Autodesk Fusion 360 part; units mm, degrees
note: some values were not read from the file. Chosen so that the rebuilt part matches the saved one: which bodies a step acts on. Set by a fixed rule: which sketch regions a step uses.
(part 2 of 2)
sketch "Sketch36" plane through (-3.3, 0, 0) normal (-1, 0, 0) x (0, -1, 0)
  line L0 (50, 42.2) -> (57.6, 42.2)
  line L1 (57.6, 42.2) -> (57.6, 27.6)
  line L2 (57.6, 27.6) -> (50, 27.6)
  line L3 (50, 27.6) -> (50, 22.6)
  line L4 (50, 22.6) -> (57.5, 22.6)
  line L5 (57.5, 22.6) -> (57.5, 8)
  line L6 (57.5, 8) -> (50, 8)
  line L7 (50, 8) -> (50, 4)
  line L8 (50, 4) -> (75, 4)
  line L9 (75, 4) -> (75, 53)
  line L10 (75, 53) -> (50, 53)
  line L11 (50, 53) -> (50, 49.75)
  line L12 (50, 49.75) -> (52, 49.75)
  line L13 (52, 49.75) -> (52, 46.25)
  line L14 (52, 46.25) -> (50, 46.25)
  line L15 (50, 46.25) -> (50, 42.2)
extrude "Extrude59" add 2 faces at (53.0448, -67, 50.2683) (4.0448, -67, 50.2683) along direction (0, 1, 0) blind 1 on bodies 3 bodies 3
extrude "Extrude60" cut 2 faces at (54.0333, -55.3333, 56.1) (2.9667, -55.3333, 56.1) along direction (0, 0, -1) blind 55.1 on bodies 3 bodies 3
sketch "Sketch37" plane through (0, -66, 0) normal (0, 1, 0) x (-1, 0, 0)
  circle A0 centre (-4, 53) radius 1.8
  line L0 (-0.9, 49.8) -> (-0.9, 56.1)
  line L1 (-0.9, 56.1) -> (-7.1, 56.1)
  line L2 (-7.1, 56.1) -> (-7.1, 49.8)
  line L3 (-7.1, 49.8) -> (-0.9, 49.8)
sketch "Sketch38" plane through (0, -66, 0) normal (0, 1, 0) x (-1, 0, 0)
  circle A0 centre (-4, 53) radius 1.8
  line L0 (-0.9, 49.8) -> (-0.9, 56.1)
  line L1 (-0.9, 56.1) -> (-7.1, 56.1)
  line L2 (-7.1, 56.1) -> (-7.1, 49.8)
  line L3 (-7.1, 49.8) -> (-0.9, 49.8)
sketch "Sketch39" plane through (0, -50, 0) normal (0, 1, 0) x (-1, 0, 0)
  line L0 (-49.9, 7.2) -> (-49.9, 1)
  line L1 (-49.9, 1) -> (-56.1, 1)
  line L2 (-56.1, 1) -> (-56.1, 7.2)
  line L3 (-56.1, 7.2) -> (-57.8, 7.2)
  line L4 (-57.8, 7.2) -> (-57.8, 15.95)
  line L5 (-57.8, 15.95) -> (-60.3, 15.95)
  line L6 (-60.3, 15.95) -> (-60.3, 4)
  arc A0 (-60.3, 4) -> (-53, -3.3) centre (-53, 4) ccw
  line L7 (-53, -3.3) -> (-4, -3.3)
  arc A1 (-4, -3.3) -> (3.3, 4) centre (-4, 4) ccw
  line L8 (3.3, 4) -> (3.3, 8)
  line L9 (3.3, 8) -> (0.8, 8)
  line L10 (0.8, 8) -> (0.8, 7.2)
  line L11 (0.8, 7.2) -> (-0.9, 7.2)
  line L12 (-0.9, 7.2) -> (-0.9, 1)
  line L13 (-0.9, 1) -> (-7.1, 1)
  line L14 (-7.1, 1) -> (-7.1, 7.2)
  line L15 (-7.1, 7.2) -> (-7.2, 7.2)
  line L16 (-7.2, 7.2) -> (-7.2, -0.8)
  line L17 (-7.2, -0.8) -> (-49.8, -0.8)
  line L18 (-49.8, -0.8) -> (-49.8, 7.2)
  line L19 (-49.8, 7.2) -> (-49.9, 7.2)
  line L20 (-0.9, 1) -> (-7.1, 1)
  line L21 (-7.1, 1) -> (-7.1, 7.2)
  line L22 (-7.1, 7.2) -> (-0.9, 7.2)
  line L23 (-0.9, 7.2) -> (-0.9, 1)
  line L24 (-56.1, 1) -> (-49.8, 1)
  line L25 (-49.8, 1) -> (-49.8, 7.2)
  line L26 (-49.8, 7.2) -> (-56.1, 7.2)
  line L27 (-56.1, 7.2) -> (-56.1, 1)
  line L28 (-0.9, 1) -> (-7.2, 1)
  line L29 (-7.2, 1) -> (-7.2, 7.2)
  line L30 (-7.2, 7.2) -> (-0.9, 7.2)
  line L31 (-0.9, 7.2) -> (-0.9, 1)
  constraint horizontal L20
  constraint vertical L21
  constraint horizontal L22
  constraint vertical L23
  constraint coincident L14.end L15.start
  constraint coincident L12.end L13.start
  constraint horizontal L24
  constraint vertical L25
  constraint horizontal L26
  constraint vertical L27
  constraint coincident L18.end L19.start
  constraint coincident L1.end L2.start
  constraint horizontal L28
  constraint vertical L29
  constraint horizontal L30
  constraint vertical L31
  constraint coincident L15.end L16.start
extrude "Extrude61" add sketch "Sketch39" against normal blind 13 contours L0 L18 L19 L24 L25 L26 | L0 L1 L2 L24 L26 L27 | L14 L15 L16 L21 L28 L29 L30 | L12 L13 L14 L20 L21 L22 L23 L28 L30 L31 bodies 3
sketch "Sketch40" plane through (0, -50, 0) normal (0, 1, 0) x (-1, 0, 0)
  line L0 (-0.9, 56.1) -> (-0.9, 49.8)
  line L1 (-0.9, 49.8) -> (0.8, 49.8)
  line L2 (0.8, 49.8) -> (0.8, 49.75)
  line L3 (0.8, 49.75) -> (3.3, 49.75)
  line L4 (3.3, 49.75) -> (3.3, 53)
  arc A0 (3.3, 53) -> (-4, 60.3) centre (-4, 53) ccw
  line L5 (-4, 60.3) -> (-53, 60.3)
  arc A1 (-53, 60.3) -> (-60.3, 53) centre (-53, 53) ccw
  line L6 (-60.3, 53) -> (-60.3, 19.45)
  line L7 (-60.3, 19.45) -> (-57.8, 19.45)
  line L8 (-57.8, 19.45) -> (-57.8, 49.8)
  line L9 (-57.8, 49.8) -> (-56.1, 49.8)
  line L10 (-56.1, 49.8) -> (-56.1, 56.1)
  line L11 (-56.1, 56.1) -> (-49.9, 56.1)
  line L12 (-49.9, 56.1) -> (-49.9, 49.8)
  line L13 (-49.9, 49.8) -> (-49.8, 49.8)
  line L14 (-49.8, 49.8) -> (-49.8, 57.8)
  line L15 (-49.8, 57.8) -> (-7.2, 57.8)
  line L16 (-7.2, 57.8) -> (-7.2, 49.8)
  line L17 (-7.2, 49.8) -> (-7.1, 49.8)
  line L18 (-7.1, 49.8) -> (-7.1, 56.1)
  line L19 (-7.1, 56.1) -> (-0.9, 56.1)
  line L20 (-56.1, 56.1) -> (-49.9, 56.1)
  line L21 (-49.9, 56.1) -> (-49.9, 49.8)
  line L22 (-49.9, 49.8) -> (-56.1, 49.8)
  line L23 (-56.1, 49.8) -> (-56.1, 56.1)
  line L24 (-0.9, 56.1) -> (-7.1, 56.1)
  line L25 (-7.1, 56.1) -> (-7.1, 49.8)
  line L26 (-7.1, 49.8) -> (-0.9, 49.8)
  line L27 (-0.9, 49.8) -> (-0.9, 56.1)
  constraint horizontal L20
  constraint vertical L21
  constraint horizontal L22
  constraint vertical L23
  constraint coincident L12.end L13.start
  constraint coincident L10.end L11.start
  constraint horizontal L24
  constraint vertical L25
  constraint horizontal L26
  constraint vertical L27
  constraint coincident L17.end L18.start
  constraint coincident L0.start L19.end
extrude "Extrude62" add sketch "Sketch40" against normal blind 13 contours L0 L18 L19 L24 L25 L26 L27 | L10 L11 L12 L20 L21 L22 L23 bodies 3
sketch "Sketch41" plane through (0, -77.5, 0) normal (0, -1, 0) x (1, 0, 0)
  circle A0 centre (4, 4) radius 1.8
  circle A1 centre (4, 53) radius 1.8
  circle A2 centre (53, 4) radius 1.8
  circle A3 centre (53, 53) radius 1.8
  circle A4 centre (39, 43.5) radius 6
  circle A5 centre (18, 43.5) radius 7
  arc A6 (-0.8, 4) -> (4, -0.8) centre (4, 4) ccw
  line L0 (4, -0.8) -> (53, -0.8)
  arc A7 (53, -0.8) -> (57.8, 4) centre (53, 4) ccw
  line L1 (57.8, 4) -> (57.8, 53)
  arc A8 (57.8, 53) -> (53, 57.8) centre (53, 53) ccw
  line L2 (53, 57.8) -> (4, 57.8)
  arc A9 (4, 57.8) -> (-0.8, 53) centre (4, 53) ccw
  line L3 (-0.8, 53) -> (-0.8, 4)
extrude "Extrude63" add sketch "Sketch41" against normal blind 3 contours A0 | A1 | A2 | A3 bodies 3
sketch "Sketch42" plane through (0, -75, 0) normal (0, 1, 0) x (-1, 0, 0)
  arc A0 (-41.1817, 55.3) -> (-27.4524, 40.2362) centre (-39, 43.5) ccw
  line L0 (-41.1817, 55.3) -> (-49.8, 55.3)
  line L1 (-49.8, 55.3) -> (-49.8, 49.8)
  line L2 (-49.8, 49.8) -> (-55.3, 49.8)
  line L3 (-55.3, 49.8) -> (-55.3, 7.2)
  line L4 (-55.3, 7.2) -> (-49.8, 7.2)
  line L5 (-49.8, 7.2) -> (-49.8, 1.7)
  line L6 (-49.8, 1.7) -> (-7.2, 1.7)
  line L7 (-7.2, 1.7) -> (-7.2, 7.2)
  line L8 (-7.2, 7.2) -> (-1.7, 7.2)
  line L9 (-1.7, 7.2) -> (-1.7, 49.8)
  line L10 (-1.7, 49.8) -> (-7.2, 49.8)
  line L11 (-7.2, 49.8) -> (-7.2, 55.3)
  line L12 (-7.2, 55.3) -> (-36.8183, 55.3)
  arc A1 (-27.4524, 46.7638) -> (-36.8183, 55.3) centre (-39, 43.5) ccw
  arc A2 (-27.4524, 40.2362) -> (-27.4524, 46.7638) centre (-18, 43.5) ccw
  line L13 (-7.2, 49.8) -> (-9.2, 49.8)
  line L14 (-9.2, 49.8) -> (-9.2, 58.8)
  line L15 (-9.2, 58.8) -> (-7.2, 58.8)
  line L16 (-7.2, 58.8) -> (-7.2, 49.8)
  line L17 (-49.8, 49.8) -> (-47.8, 49.8)
  line L18 (-47.8, 49.8) -> (-47.8, 58.8)
  line L19 (-47.8, 58.8) -> (-49.8, 58.8)
  line L20 (-49.8, 58.8) -> (-49.8, 49.8)
  dimension "d264" = 2
  dimension "d265" = 9
  dimension "d266" = 2
  dimension "d267" = 9
  constraint horizontal L13
  constraint vertical L14
  constraint horizontal L15
  constraint vertical L16
  constraint coincident L10.end L11.start
  constraint horizontal L17
  constraint vertical L18
  constraint horizontal L19
  constraint vertical L20
  constraint coincident L1.end L2.start
  measures "d264" distance of L10.end L13.end
  measures "d265" distance of L10.end L15.end
  measures "d266" distance of L1.end L17.end
  measures "d267" distance of L1.end L19.end
extrude "Extrude64" add sketch "Sketch42" along normal blind 13 contours A0 L17 L18 | A0 L0 L1 L17 L18 L20 | L0 L18 L19 L20 | L12 L14 L15 L16 | L11 L12 L13 L14 L16 bodies 3
sketch "Sketch43" plane through (0, -75, 0) normal (0, 1, 0) x (-1, 0, 0)
  line L0 (-1.7, 49.8) -> (-9.2, 49.8)
  line L1 (-9.2, 49.8) -> (-9.2, 55.3)
  line L2 (-9.2, 55.3) -> (-36.8183, 55.3)
  arc A0 (-27.4524, 46.7638) -> (-36.8183, 55.3) centre (-39, 43.5) ccw
  arc A1 (-27.4524, 40.2362) -> (-27.4524, 46.7638) centre (-18, 43.5) ccw
  arc A2 (-49.2132, 49.8) -> (-27.4524, 40.2362) centre (-39, 43.5) ccw
  line L3 (-49.2132, 49.8) -> (-55.3, 49.8)
  line L4 (-55.3, 49.8) -> (-55.3, 7.2)
  line L5 (-55.3, 7.2) -> (-49.8, 7.2)
  line L6 (-49.8, 7.2) -> (-49.8, 1.7)
  line L7 (-49.8, 1.7) -> (-7.2, 1.7)
  line L8 (-7.2, 1.7) -> (-7.2, 7.2)
  line L9 (-7.2, 7.2) -> (-1.7, 7.2)
  line L10 (-1.7, 7.2) -> (-1.7, 49.8)
  line L11 (-7.2, 7.2) -> (-9.2, 7.2)
  line L12 (-9.2, 7.2) -> (-9.2, -1.8)
  line L13 (-9.2, -1.8) -> (-7.2, -1.8)
  line L14 (-7.2, -1.8) -> (-7.2, 7.2)
  line L15 (-49.8, 7.2) -> (-47.8, 7.2)
  line L16 (-47.8, 7.2) -> (-47.8, -1.8)
  line L17 (-47.8, -1.8) -> (-49.8, -1.8)
  line L18 (-49.8, -1.8) -> (-49.8, 7.2)
  dimension "d270" = 2
  dimension "d271" = 9
  dimension "d272" = 2
  dimension "d273" = 9
  constraint horizontal L11
  constraint vertical L12
  constraint horizontal L13
  constraint vertical L14
  constraint coincident L8.end L9.start
  constraint horizontal L15
  constraint vertical L16
  constraint horizontal L17
  constraint vertical L18
  constraint coincident L5.end L6.start
  measures "d270" distance of L8.end L11.end
  measures "d271" distance of L8.end L13.end
  measures "d272" distance of L5.end L15.end
  measures "d273" distance of L5.end L17.end
extrude "Extrude65" add sketch "Sketch43" along normal blind 13 contours L7 L8 L11 L12 L14 | L7 L12 L13 L14 | L7 L16 L17 L18 | L6 L7 L15 L16 L18 bodies 3
sketch "Sketch44" plane through (0, 1.25, 0) normal (0, -1, 0) x (1, 0, 0)
  circle A0 centre (4, 4) radius 1.8
  circle A1 centre (4, 53) radius 1.8
  circle A2 centre (53, 4) radius 1.8
  circle A3 centre (53, 53) radius 1.8
  line L0 (21.9074, 57.8) -> (21.9074, 55.8)
  line L1 (21.9074, 55.8) -> (49.8, 55.8)
  line L2 (49.8, 55.8) -> (49.8, 49.8)
  line L3 (49.8, 49.8) -> (55.8, 49.8)
  line L4 (55.8, 49.8) -> (55.8, 7.2)
  line L5 (55.8, 7.2) -> (49.8, 7.2)
  line L6 (49.8, 7.2) -> (49.8, 1.2)
  line L7 (49.8, 1.2) -> (7.2, 1.2)
  line L8 (7.2, 1.2) -> (7.2, 7.2)
  line L9 (7.2, 7.2) -> (1.2, 7.2)
  line L10 (1.2, 7.2) -> (1.2, 49.8)
  line L11 (1.2, 49.8) -> (7.2, 49.8)
  line L12 (7.2, 49.8) -> (7.2, 57.8)
  line L13 (7.2, 57.8) -> (4, 57.8)
  arc A4 (4, 57.8) -> (-0.8, 53) centre (4, 53) ccw
  line L14 (-0.8, 53) -> (-0.8, 4)
  arc A5 (-0.8, 4) -> (4, -0.8) centre (4, 4) ccw
  line L15 (4, -0.8) -> (53, -0.8)
  arc A6 (53, -0.8) -> (57.8, 4) centre (53, 4) ccw
  line L16 (57.8, 4) -> (57.8, 53)
  arc A7 (57.8, 53) -> (53, 57.8) centre (53, 53) ccw
  line L17 (53, 57.8) -> (21.9074, 57.8)
sketch "Sketch45" plane through (0, 1.25, 0) normal (0, -1, 0) x (1, 0, 0)
  circle A0 centre (4, 4) radius 1.8
  circle A1 centre (4, 53) radius 1.8
  circle A2 centre (53, 4) radius 1.8
  circle A3 centre (53, 53) radius 1.8
  line L0 (21.9074, 57.8) -> (21.9074, 55.8)
  line L1 (21.9074, 55.8) -> (49.8, 55.8)
  line L2 (49.8, 55.8) -> (49.8, 49.8)
  line L3 (49.8, 49.8) -> (55.8, 49.8)
  line L4 (55.8, 49.8) -> (55.8, 7.2)
  line L5 (55.8, 7.2) -> (49.8, 7.2)
  line L6 (49.8, 7.2) -> (49.8, 1.2)
  line L7 (49.8, 1.2) -> (7.2, 1.2)
  line L8 (7.2, 1.2) -> (7.2, 7.2)
  line L9 (7.2, 7.2) -> (1.2, 7.2)
  line L10 (1.2, 7.2) -> (1.2, 49.8)
  line L11 (1.2, 49.8) -> (7.2, 49.8)
  line L12 (7.2, 49.8) -> (7.2, 57.8)
  line L13 (7.2, 57.8) -> (4, 57.8)
  arc A4 (4, 57.8) -> (-0.8, 53) centre (4, 53) ccw
  line L14 (-0.8, 53) -> (-0.8, 4)
  arc A5 (-0.8, 4) -> (4, -0.8) centre (4, 4) ccw
  line L15 (4, -0.8) -> (53, -0.8)
  arc A6 (53, -0.8) -> (57.8, 4) centre (53, 4) ccw
  line L16 (57.8, 4) -> (57.8, 53)
  arc A7 (57.8, 53) -> (53, 57.8) centre (53, 53) ccw
  line L17 (53, 57.8) -> (21.9074, 57.8)
sketch "Sketch46" plane through (0, 1.25, 0) normal (0, -1, 0) x (1, 0, 0)
  circle A0 centre (4, 4) radius 1.8
  circle A1 centre (4, 53) radius 1.8
  circle A2 centre (53, 4) radius 1.8
  circle A3 centre (53, 53) radius 1.8
  line L0 (21.9074, 57.8) -> (21.9074, 55.8)
  line L1 (21.9074, 55.8) -> (49.8, 55.8)
  line L2 (49.8, 55.8) -> (49.8, 49.8)
  line L3 (49.8, 49.8) -> (55.8, 49.8)
  line L4 (55.8, 49.8) -> (55.8, 7.2)
  line L5 (55.8, 7.2) -> (49.8, 7.2)
  line L6 (49.8, 7.2) -> (49.8, 1.2)
  line L7 (49.8, 1.2) -> (7.2, 1.2)
  line L8 (7.2, 1.2) -> (7.2, 7.2)
  line L9 (7.2, 7.2) -> (1.2, 7.2)
  line L10 (1.2, 7.2) -> (1.2, 49.8)
  line L11 (1.2, 49.8) -> (7.2, 49.8)
  line L12 (7.2, 49.8) -> (7.2, 57.8)
  line L13 (7.2, 57.8) -> (4, 57.8)
  arc A4 (4, 57.8) -> (-0.8, 53) centre (4, 53) ccw
  line L14 (-0.8, 53) -> (-0.8, 4)
  arc A5 (-0.8, 4) -> (4, -0.8) centre (4, 4) ccw
  line L15 (4, -0.8) -> (53, -0.8)
  arc A6 (53, -0.8) -> (57.8, 4) centre (53, 4) ccw
  line L16 (57.8, 4) -> (57.8, 53)
  arc A7 (57.8, 53) -> (53, 57.8) centre (53, 53) ccw
  line L17 (53, 57.8) -> (21.9074, 57.8)
  circle A8 centre (4, 4) radius 1.55
  circle A9 centre (53, 4) radius 1.55
  circle A10 centre (53, 53) radius 1.55
  circle A11 centre (4, 53) radius 1.55
  circle A12 centre (53, 53) radius 1.8
  circle A13 centre (4, 53) radius 1.8
  circle A14 centre (4, 4) radius 1.8
  circle A15 centre (53, 4) radius 1.8
  dimension "d276" = 3.1
  dimension "d277" = 3.1
  dimension "d278" = 3.1
  dimension "d279" = 3.1
  constraint concentric A0 A8
  constraint concentric A2 A9
  constraint concentric A3 A10
  constraint concentric A1 A11
  constraint concentric A3 A12
  constraint concentric A1 A13
  constraint concentric A0 A14
  constraint concentric A9 A15
  measures "d276" diameter of A8
  measures "d277" diameter of A9
  measures "d278" diameter of A10
  measures "d279" diameter of A11
extrude "Extrude66" add sketch "Sketch46" against normal blind 6.25 contours A0 A14 | A1 A13 | A2 A15 | A3 A12 bodies 2
sketch "Sketch47" plane through (0, 12.5, 0) normal (0, 1, 0) x (-1, 0, 0)
  circle A0 centre (-4, 53) radius 3.25
  circle A1 centre (-4, 4) radius 3.25
  circle A2 centre (-53, 53) radius 3.25
  circle A3 centre (-53, 4) radius 3.25
  line L0 (-4, 60.3) -> (-53, 60.3)
  arc A4 (-53, 60.3) -> (-60.3, 53) centre (-53, 53) ccw
  line L1 (-60.3, 53) -> (-60.3, 4)
  arc A5 (-60.3, 4) -> (-53, -3.3) centre (-53, 4) ccw
  line L2 (-53, -3.3) -> (-4, -3.3)
  arc A6 (-4, -3.3) -> (3.3, 4) centre (-4, 4) ccw
  line L3 (3.3, 4) -> (3.3, 53)
  arc A7 (3.3, 53) -> (-4, 60.3) centre (-4, 53) ccw
  circle A8 centre (-4, 4) radius 1.55
  circle A9 centre (-53, 4) radius 1.55
  circle A10 centre (-53, 53) radius 1.55
  circle A11 centre (-4, 53) radius 1.55
  dimension "d282" = 3.1
  dimension "d283" = 3.1
  dimension "d284" = 3.1
  dimension "d285" = 3.1
  constraint concentric A1 A8
  constraint concentric A3 A9
  constraint concentric A2 A10
  constraint concentric A0 A11
  measures "d282" diameter of A8
  measures "d283" diameter of A9
  measures "d284" diameter of A10
  measures "d285" diameter of A11
extrude "Extrude67" cut sketch "Sketch47" against normal blind 77 contours A8 | A9 | A10 | A11 bodies 3
extrude "Extrude68" add 1 faces at (31.0558, -65, 42.7548) along direction (0, 1, 0) blind 8 on bodies 3 bodies 3
sketch "Sketch48" plane through (0, -57, 0) normal (0, 1, 0) x (-1, 0, 0)
  circle A0 centre (-39, 43.5) radius 9
  circle A1 centre (-39, 43.5) radius 6
  circle A2 centre (-39, 43.5) radius 6
  constraint concentric A0 A2
extrude "Extrude69" add sketch "Sketch48" against normal blind 2 contours A1 A2 bodies 3
sketch "Sketch49" plane through (0, -59, 0) normal (0, -1, 0) x (1, 0, 0)
  circle A0 centre (39, 43.5) radius 6
  circle A1 centre (39, 43.5) radius 3.5
  circle A2 centre (39, 43.5) radius 2.369
  dimension "d292" = 7
  constraint concentric A0 A1
  constraint concentric A1 A2
  measures "d292" diameter of A1
extrude "Extrude70" cut sketch "Sketch49" against normal blind 4 contours A1 | A2 bodies 3
fillet "Fillet8" radius 5.5 1 edges at (33.406, -59, 45.6697) on bodies 3
fillet "Fillet9" radius 1.5 1 edges at (7.2, -62, 53.8) on bodies 3
fillet "Fillet10" radius 2 3 edges at (49.8, -62, 53.8) (49.8, -62, 3.2) (7.2, -62, 3.2) on bodies 3
sketch "Sketch50" plane through (0, -77.5, 0) normal (0, -1, 0) x (1, 0, 0)
  circle A0 centre (39, 43.5) radius 6
  circle A1 centre (18, 43.5) radius 7
  arc A2 (-0.8, 4) -> (4, -0.8) centre (4, 4) ccw
  line L0 (4, -0.8) -> (53, -0.8)
  arc A3 (53, -0.8) -> (57.8, 4) centre (53, 4) ccw
  line L1 (57.8, 4) -> (57.8, 53)
  arc A4 (57.8, 53) -> (53, 57.8) centre (53, 53) ccw
  line L2 (53, 57.8) -> (4, 57.8)
  arc A5 (4, 57.8) -> (-0.8, 53) centre (4, 53) ccw
  line L3 (-0.8, 53) -> (-0.8, 4)
extrude "Extrude71" add sketch "Sketch50" along normal blind 15 separate body contours A1 makes body 6
sketch "Sketch51" plane through (0, -92.5, 0) normal (0, -1, 0) x (1, 0, 0)
  circle A0 centre (18, 43.5) radius 7
  circle A1 centre (18, 43.5) radius 1.3957
  circle A2 centre (18, 43.5) radius 3.297
  constraint concentric A0 A1
  constraint concentric A1 A2
extrude "Extrude72" cut sketch "Sketch51" against normal blind 11 contours A1 | A2 bodies 6
move_body "Move3" bodies 1 to x (1, 0, 0) y (0, 1, 0) z (0, 0, 1) at (0, 20, 0)
move_body "Move4" bodies 3 to x (1, 0, 0) y (0, 1, 0) z (0, 0, 1) at (0, 50, 0)
move_body "Move5" bodies 6 to x (1, 0, 0) y (0, 1, 0) z (0, 0, 1) at (0, 50, 0)
sketch "Sketch52" plane through (0, 0, 60.3) normal (0, 0, 1) x (-1, 0, 0)
  circle A0 centre (-11.43, 8.81) radius 3
  line L0 (-4, 25) -> (-53, 25)
  line L1 (-53, 25) -> (-53, 0)
  line L2 (-53, 0) -> (-4, 0)
  line L3 (-4, 0) -> (-4, 25)
extrude "Extrude73" add sketch "Sketch52" along normal blind 10 separate body contours A0 makes body 7
sketch "Sketch53" plane through (0, -31.5, 0) normal (0, -1, 0) x (1, 0, 0)
  circle A0 centre (18, 43.5) radius 3.297
  circle A1 centre (18, 43.5) radius 2.7993
  constraint concentric A0 A1
extrude "Extrude74" add sketch "Sketch53" 1 faces at (16.4003, -31.5, 44.3672) along normal blind 6 contours A1 on bodies 6 bodies 6
sketch "Sketch54" plane through (0, 9.5, 0) normal (0, -1, 0) x (1, 0, 0)
  line L0 (9.7, 9.7) -> (9.7, 1.2)
  line L1 (9.7, 1.2) -> (47.3, 1.2)
  line L2 (47.3, 1.2) -> (47.3, 9.7)
  line L3 (47.3, 9.7) -> (55.8, 9.7)
  line L4 (55.8, 9.7) -> (55.8, 47.3)
  line L5 (55.8, 47.3) -> (47.3, 47.3)
  line L6 (47.3, 47.3) -> (47.3, 55.8)
  line L7 (47.3, 55.8) -> (9.7, 55.8)
  line L8 (9.7, 55.8) -> (9.7, 47.3)
  line L9 (9.7, 47.3) -> (1.2, 47.3)
  line L10 (1.2, 47.3) -> (1.2, 9.7)
  line L11 (1.2, 9.7) -> (9.7, 9.7)
  circle A0 centre (38.9991, 43.5419) radius 3.0067
extrude "Extrude75" add sketch "Sketch49" along normal blind 6 contours A2 bodies 3 makes body 8
move_body "Move6" bodies 8 to x (1, 0, 0) y (0, 1, 0) z (0, 0, 1) at (0, 59, 0)
sketch "Sketch55" plane through (-3.3, 0, 0) normal (-1, 0, 0) x (0, -1, 0)
  line L0 (0, 42.2) -> (7.6, 42.2)
  line L1 (7.6, 42.2) -> (7.6, 27.6)
  line L2 (7.6, 27.6) -> (0, 27.6)
  line L3 (0, 27.6) -> (0, 22.6)
  line L4 (0, 22.6) -> (7.5, 22.6)
  line L5 (7.5, 22.6) -> (7.5, 8)
  line L6 (7.5, 8) -> (0, 8)
  line L7 (0, 8) -> (0, 4)
  line L8 (0, 4) -> (25, 4)
  line L9 (25, 4) -> (25, 53)
  line L10 (25, 53) -> (0, 53)
  line L11 (0, 53) -> (0, 49.75)
  line L12 (0, 49.75) -> (2, 49.75)
  line L13 (2, 49.75) -> (2, 46.25)
  line L14 (2, 46.25) -> (0, 46.25)
  line L15 (0, 46.25) -> (0, 42.2)
  line L16 (0, 42) -> (7.6, 42)
  line L17 (7.6, 42) -> (7.6, 27.6)
  line L18 (7.6, 27.6) -> (0, 27.6)
  line L19 (0, 27.6) -> (0, 42)
  line L20 (0.4121, 22.6) -> (7.5, 22.6)
  line L21 (7.5, 22.6) -> (7.5, 8)
  line L22 (7.5, 8) -> (0.4121, 8)
  line L23 (0.4121, 8) -> (0.4121, 22.6)
  constraint horizontal L16
  constraint vertical L17
  constraint horizontal L18
  constraint vertical L19
  constraint coincident L1.end L2.start
  constraint horizontal L20
  constraint vertical L21
  constraint horizontal L22
  constraint vertical L23
  constraint coincident L5.end L6.start
  constraint coincident L4 L20.start
sketch "Sketch56" plane through (-3.3, 0, 0) normal (-1, 0, 0) x (0, -1, 0)
  line L0 (0, 42.2) -> (7.6, 42.2)
  line L1 (7.6, 42.2) -> (7.6, 27.6)
  line L2 (7.6, 27.6) -> (0, 27.6)
  line L3 (0, 27.6) -> (0, 22.6)
  line L4 (0, 22.6) -> (7.5, 22.6)
  line L5 (7.5, 22.6) -> (7.5, 8)
  line L6 (7.5, 8) -> (0, 8)
  line L7 (0, 8) -> (0, 4)
  line L8 (0, 4) -> (25, 4)
  line L9 (25, 4) -> (25, 53)
  line L10 (25, 53) -> (0, 53)
  line L11 (0, 53) -> (0, 49.75)
  line L12 (0, 49.75) -> (2, 49.75)
  line L13 (2, 49.75) -> (2, 46.25)
  line L14 (2, 46.25) -> (0, 46.25)
  line L15 (0, 46.25) -> (0, 42.2)
extrude "Extrude76" add sketch "Sketch55" along normal blind 0.1 separate body contours L1 L2 L16 L17 L18 L19 | L4 L5 L6 L20 L21 L22 L23 makes body 9 at (-3.3, -2.5333, 37.2) makes body 10 at (-3.3, -2.7747, 12.8667)
copy_body "CopyPasteBodies1" bodies 3 7 10 1 8 6 9 2 makes body 11 makes body 12 makes body 13 makes body 14 makes body 15 makes body 16 makes body 17 makes body 18
move_body "Move7" bodies 11 12 13 14 15 16 17 18 to x (-1, 0, 0) y (0, -1, 0) z (0, 0, 1) at (56.4, -195, 0)
sketch "Sketch57" plane through (0, 0, -3.3) normal (0, 0, -1) x (1, 0, 0)
  line L0 (53, 25) -> (4, 25)
  line L1 (4, 25) -> (4, 0)
  line L2 (4, 0) -> (53, 0)
  line L3 (53, 0) -> (53, 25)
  line L4 (-3.2283, -12.3465) -> (5.4051, -12.3465)
  line L5 (5.4051, -12.3465) -> (5.4051, -51.3017)
  line L6 (5.4051, -51.3017) -> (-3.2283, -51.3017)
  line L7 (-3.2283, -51.3017) -> (-3.2283, -12.3465)
  line L8 (-3.2283, -51.3017) -> (126.4124, -51.3017)
  line L9 (126.4124, -51.3017) -> (126.4124, 265.7054)
  line L10 (126.4124, 265.7054) -> (-3.2283, 265.7054)
  line L11 (-3.2283, 265.7054) -> (-3.2283, -51.3017)
  constraint horizontal L4
  constraint vertical L5
  constraint horizontal L6
  constraint vertical L7
  constraint horizontal L8
  constraint vertical L9
  constraint horizontal L10
  constraint vertical L11
extrude "Extrude77" add sketch "Sketch57" along normal blind 10 contours L4 L5 L8 L9 L10 L11 bodies 2 6 7 9 10 12 13 14 16 17 3 11 18
extrude "Extrude78" add 1 faces at (5.4051, 25.3827, -9.9667) along direction (-1, 0, 0) blind 9 on bodies 2 bodies 2
extrude "Extrude79" cut 1 faces at (-3.3505, 12.3465, -6.6333) along direction (0, 1, 0) blind 62 on bodies 2 bodies 2
split "Split1" by plane through (5.4051, 12.3465, -3.3) normal (0, 0, 1) bodies 2 makes body 19 at (35.2725, -207.5, 21.0702) makes body 20 at (21.1275, 12.5, 21.0702)
extrude "Extrude80" add 1 faces at (126.4124, -54.3673, -6.6333) along direction (1, 0, 0) blind 360 on bodies 2 bodies 2
extrude "Extrude81" add 1 faces at (323.1988, 51.3017, -9.9667) along direction (0, 1, 0) blind 525 on bodies 2 bodies 2
extrude "Extrude82" add 1 faces at (323.1988, -265.7054, -6.6333) along direction (0, -1, 0) blind 340 on bodies 2 bodies 2
move_body "Move8" bodies 2 to x (1, 0, 0) y (0, 1, 0) z (0, 0, 1) at (-170, 0, 0)
extrude "Extrude1" [suppressed]
extrude "Extrude2" [suppressed]
extrude "Extrude3" [suppressed]
sketch "Sketch2" plane through (0, 20, 0) normal (0, 1, 0) x (-1, 0, 0)
  arc A0 (-53, 57.8) -> (-57.8, 53) centre (-53, 53) ccw
  line L0 (-53, 57.8) -> (-4, 57.8)
  arc A1 (0.8, 53) -> (-4, 57.8) centre (-4, 53) ccw
  line L1 (0.8, 53) -> (0.8, 4)
  arc A2 (-4, -0.8) -> (0.8, 4) centre (-4, 4) ccw
  line L2 (-4, -0.8) -> (-53, -0.8)
  arc A3 (-57.8, 4) -> (-53, -0.8) centre (-53, 4) ccw
  line L3 (-57.8, 4) -> (-57.8, 53)
  arc A4 (-53, 60.3) -> (-60.3, 53) centre (-53, 53) ccw
  line L4 (-60.3, 53) -> (-60.3, 4)
  arc A5 (-60.3, 4) -> (-53, -3.3) centre (-53, 4) ccw
  line L5 (-53, -3.3) -> (-4, -3.3)
  arc A6 (-4, -3.3) -> (3.3, 4) centre (-4, 4) ccw
  line L6 (3.3, 4) -> (3.3, 53)
  arc A7 (3.3, 53) -> (-4, 60.3) centre (-4, 53) ccw
  line L7 (-4, 60.3) -> (-53, 60.3)
extrude "Extrude4" [suppressed]
fillet "Fillet1" [suppressed]
fillet "Fillet2" [suppressed]
extrude "Extrude5" [suppressed]
sketch "Sketch3" plane through (0.5, 0, 0) normal (-1, 0, 0) x (0, -1, 0)
  line L0 (0, 47) -> (0, 49)
  line L1 (0, 49) -> (-1, 49)
  line L2 (-1, 49) -> (-1, 47)
  line L3 (-1, 47) -> (0, 47)
extrude "Extrude6" [suppressed]
hidden bodies 2
equation "d256 = 48.9 mm + 6.2 mm"
